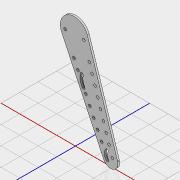
# Autodesk Inventor part: ЛЦМК.30000.30.00.02 Штанга
Saved by Autodesk Inventor 2021.2 (Build 252289000, 289)
## iProperties
Created: 2025-11-10
Part Number: ЛЦМК.30000.30.00.02 Штанга
Material: Типовые
Document SubType Name: Modeling
Designer: Захаров
Density: 1 g/cm^3
Appearance: По умолчанию
Mass: 8.66485 g
Surface Area: 67.4895 cm^2
Volume: 8.66485 cm^3
Author: Захаров
Autodesk Inventor part; units mm, degrees
ref_plane "YZ Plane" through (0, 0, 0) normal (1, 0, 0) x (0, 1, 0)
ref_plane "XZ Plane" through (0, 0, 0) normal (0, 1, 0) x (-1, 0, 0)
ref_plane "XY Plane" through (0, 0, 0) normal (0, 0, 1) x (1, 0, 0)
sketch "Эскиз1" plane through (0, 0, 0) normal (0, 0, 1) x (1, 0, 0)
  line L0 (15, -22.25) -> (15, 22.25) projected
  line L1 (15, 22.25) -> (-20, 22.25) projected
  line L2 (-20, 22.25) -> (-20, -22.25) projected
  line L3 (-20, -22.25) -> (15, -22.25) projected
  circle A0 centre (8.763, 2.3275) radius 1.5 projected
  circle A1 centre (8.763, 7.3275) radius 1.5 projected
  circle A2 centre (-11.237, -7.6725) radius 1.5 projected
  circle A3 centre (-11.237, -2.6725) radius 1.5 projected
  circle A4 centre (8.763, -2.6725) radius 1.5 projected
  circle A5 centre (8.763, -7.6725) radius 1.5 projected
  circle A6 centre (-11.237, 2.3275) radius 1.5 projected
  circle A7 centre (-11.237, 7.3275) radius 1.5 projected
  line L4 (-25, 92.25) -> (-62.0049, 92.25) projected
  line L5 (-103.637, 92.25) -> (-67.893, 92.25) projected
  circle A8 centre (-49, 104.25) radius 1.5 projected
  circle A9 centre (-42, 104.25) radius 1.5 projected
  circle A10 centre (-35, 104.25) radius 1.5 projected
  circle A11 centre (-35, 111.25) radius 1.5 projected
  circle A12 centre (-42, 118.25) radius 1.5 projected
  circle A13 centre (-49, 118.25) radius 1.5 projected
  circle A14 centre (-49, 111.25) radius 1.5 projected
  circle A15 centre (-35, 118.25) radius 1.5 projected
  circle A16 centre (-42, 111.25) radius 1.5 projected
  circle A17 centre (-42, 97.25) radius 1.5 projected
  circle A18 centre (-35, 97.25) radius 1.5 projected
  circle A19 centre (-49, 97.25) radius 1.5 projected
  line L6 (-25, 92.25) -> (-62.0049, 92.25) projected
  line L7 (-25, 95.25) -> (-25, 92.25) projected
  line L8 (-20, 95.25) -> (-25, 95.25) projected
  line L9 (-20, 95.25) -> (-20, 123.25) projected
  line L10 (-28, 123.25) -> (-20, 123.25) projected
  line L11 (-28, 129.25) -> (-28, 123.25) projected
  line L12 (-28, 129.25) -> (-62.0049, 129.25) projected
  line L13 (-62.0049, 92.25) -> (-62.0049, 129.25) projected
  line L14 (-5.1452, 11.625) -> (-40, 100) construction
  arc A20 (-32.5697, 102.9649) -> (-47.4303, 97.0351) centre (-40, 100) ccw
  line L15 (-5.1452, 11.625) -> (-22.5726, 55.8125) construction
  arc A21 (-13.8135, 8.0713) -> (-4.3725, 15.1785) centre (-0.8009, 0.6099) ccw
  line L16 (12.7625, 7.0157) -> (-32.7662, 103.4164)
  line L17 (-47.6184, 97.5588) -> (-15.0854, -3.9674)
  point P0 (0, 0)
  point P1 (-13.8589, 33.7187)
  point P2 (-33.6095, 104.8127)
  point P3 (-34.2206, 105.5316)
  point P4 (-47.7749, 98.1155)
  point P5 (-47.5011, 97.1926)
  dimension "d0" = 8
  dimension "d1" = 95
  dimension "d2" = 100
  dimension "d3" = 40
  dimension "d4" = 15
  constraints: 12 end point, 8 point on circle, 4 tangent, 2 centre point, 2 midpoint, 1 point on line
  measures "d0" radius of A20
  measures "d1" distance of L14.start L14.end
  measures "d2" vertical distance of point (0, 0) L14.end
  measures "d3" horizontal distance of point (0, 0) L14.end
  measures "d4" radius of A21
extrude "Выдавливание1" add sketch "Эскиз1" along normal blind 2 contours L16 A21 L17 L2 L1 | L1 L2 L17 L4 L16 | L4 L17 A19 A20 A10 L16 | A20 A10 | A10 A20 | A1 | A2 | A3 | A4 | A5 | A7 | A9
sketch "Эскиз2" plane through (0, 0, 2) normal (0, 0, 1) x (1, 0, 0)
  circle A0 centre (-38.5661, 86.5462) radius 1.5
  line L0 (-47.5011, 97.1926) -> (-15.0854, -3.9674) projected
  circle A1 centre (-35.5146, 77.0232) radius 1.5
  circle A2 centre (-32.463, 67.5001) radius 1.5
  circle A3 centre (-29.4114, 57.9771) radius 1.5
  circle A4 centre (-26.3599, 48.4541) radius 1.5
  circle A5 centre (-23.3083, 38.9311) radius 1.5
  circle A6 centre (-20.2568, 29.408) radius 1.5
  circle A7 centre (-17.2052, 19.885) radius 1.5
  circle A8 centre (-42, 97.25) radius 1.5 projected
  circle A9 centre (-11.237, 2.3275) radius 1.5 projected
  point P0 (0, 0)
  dimension "d7" = 3
  dimension "d10" = 10
  dimension "d17" = 5.2562
  dimension "d18" = 5.26
  constraints: 8 centre point, 15 other
  measures "d7" diameter of A0
  measures "d10" distance of A0.centre A1.centre
  measures "d17" distance from line of L0 A8.centre
  measures "d18" distance from line of L0 A0.centre
extrude "Выдавливание2" cut sketch "Эскиз2" against normal blind 3 contours A0 | A1 | A2 | A3 | A4 | A5 | A6 | A7
sketch "Эскиз3" plane through (0, 0, 2) normal (0, 0, 1) x (1, 0, 0)
  circle A0 centre (-35, 97.25) radius 1.5 projected
  line L0 (12.7625, 7.0157) -> (-32.7662, 103.4164) projected
  circle A1 centre (-30.5318, 87.7899) radius 1.5
  circle A2 centre (-26.2613, 78.7476) radius 1.5
  circle A3 centre (-21.9908, 69.7054) radius 1.5
  circle A4 centre (-17.7202, 60.6631) radius 1.5
  circle A5 centre (-13.4497, 51.6208) radius 1.5
  circle A6 centre (-9.1792, 42.5786) radius 1.5
  circle A7 centre (-4.9086, 33.5363) radius 1.5
  circle A8 centre (-0.6381, 24.494) radius 1.5
  point P0 (0, 0)
  dimension "d19" = 3
  dimension "d20" = 4.6533
  dimension "d21" = 4.653
  dimension "d24" = 10
  constraints: 8 centre point, 15 other
  measures "d19" diameter of A1
  measures "d20" distance from line of L0 A0.centre
  measures "d21" distance from line of L0 A1.centre
  measures "d24" distance of A1.centre A2.centre
extrude "Выдавливание3" cut sketch "Эскиз3" against normal blind 3 contours A1 | A2 | A3 | A4 | A5 | A6 | A7 | A8
sketch "Эскиз4" plane through (0, 0, 0) normal (0, 0, -1) x (-1, 0, 0)
  circle A0 centre (42, 97.25) radius 1.5 projected
  circle A1 centre (35, 97.25) radius 1.5 construction
  arc A2 (35, 97.25) -> (36.2942, 93.1949) centre (42, 97.25) ccw construction
  arc A3 (33.5, 97.25) -> (35.0715, 92.326) centre (42, 97.25) ccw
  arc A4 (36.5, 97.25) -> (37.5169, 94.0639) centre (42, 97.25) ccw
  arc A5 (36.5, 97.25) -> (33.5, 97.25) centre (35, 97.25) ccw construction
  arc A6 (35.0715, 92.326) -> (37.5169, 94.0639) centre (36.2942, 93.1949) ccw
  arc A7 (36.7604, 101.8918) -> (35.0715, 96.252) centre (42, 97.25) ccw construction
  arc A8 (35.6376, 102.8865) -> (33.5868, 96.0382) centre (42, 97.25) ccw
  arc A9 (37.8832, 100.8971) -> (36.5562, 96.4659) centre (42, 97.25) ccw
  arc A10 (37.8832, 100.8971) -> (35.6376, 102.8865) centre (36.7604, 101.8918) ccw
  arc A11 (33.5868, 96.0382) -> (36.5562, 96.4659) centre (35.0715, 96.252) ccw construction
  point P0 (0, 0)
  constraints: 21 point on circle, 10 centre point, 8 tangent, 2 coincident, 2 concentric
extrude "Выдавливание4" cut sketch "Эскиз4" against normal blind 3 contours A8 A10 A9 A4 A6 A3
sketch "Эскиз5" plane through (0, 0, 2) normal (0, 0, 1) x (1, 0, 0)
  circle A0 centre (-42, 97.25) radius 1.5 projected
  circle A1 centre (-11.237, 2.3275) radius 1.5 projected
  circle A2 centre (8.763, 2.3275) radius 1.5 projected
  arc A3 (-15.0854, -3.9674) -> (12.7625, 7.0157) centre (-0.8009, 0.6099) ccw projected
  line L0 (12.7625, 7.0157) -> (-32.7662, 103.4164) projected
  arc A4 (-32.7662, 103.4164) -> (-33.6095, 104.8127) centre (-40, 100) ccw projected
  arc A5 (-33.6095, 104.8127) -> (-34.2206, 105.5316) centre (-35, 104.25) ccw projected
  arc A6 (-34.2206, 105.5316) -> (-47.7749, 98.1155) centre (-40, 100) ccw projected
  arc A7 (-47.5011, 97.1926) -> (-47.7749, 98.1155) centre (-49, 97.25) ccw projected
  line L1 (-47.5011, 97.1926) -> (-15.0854, -3.9674) projected
  circle A8 centre (-17.2052, 19.885) radius 1.5 projected
  circle A9 centre (-23.3083, 38.9311) radius 1.5 projected
  circle A10 centre (-38.5661, 86.5462) radius 1.5 projected
  circle A11 centre (-32.463, 67.5001) radius 1.5 projected
  circle A12 centre (-29.4114, 57.9771) radius 1.5 projected
  circle A13 centre (-35.5146, 77.0232) radius 1.5 projected
  circle A14 centre (-20.2568, 29.408) radius 1.5 projected
  circle A15 centre (-26.3599, 48.4541) radius 1.5 projected
  circle A16 centre (-0.6381, 24.494) radius 1.5 projected
  circle A17 centre (-26.2613, 78.7476) radius 1.5 projected
  circle A18 centre (-4.9086, 33.5363) radius 1.5 projected
  circle A19 centre (-13.4497, 51.6208) radius 1.5 projected
  circle A20 centre (-17.7202, 60.6631) radius 1.5 projected
  circle A21 centre (-9.1792, 42.5786) radius 1.5 projected
  circle A22 centre (-30.5318, 87.7899) radius 1.5 projected
  circle A23 centre (-21.9908, 69.7054) radius 1.5 projected
  circle A24 centre (-23.3083, 38.9311) radius 1.5 projected
  circle A25 centre (-9.1792, 42.5786) radius 1.5 projected
  arc A26 (-9.149, 35.4026) -> (-9.1792, 42.5786) centre (-23.3083, 38.9311) ccw construction
  arc A27 (-7.6935, 35.0399) -> (-7.7268, 42.9535) centre (-23.3083, 38.9311) ccw
  arc A28 (-10.6045, 35.7653) -> (-10.6316, 42.2036) centre (-23.3083, 38.9311) ccw
  arc A29 (-10.6045, 35.7653) -> (-7.6935, 35.0399) centre (-9.149, 35.4026) ccw
  arc A30 (-7.7268, 42.9535) -> (-10.6316, 42.2036) centre (-9.1792, 42.5786) ccw
  arc A31 (-9.1792, 42.5786) -> (-11.0829, 46.8983) centre (-23.3083, 38.9311) ccw construction
  arc A32 (-7.7268, 42.9535) -> (-9.8263, 47.7173) centre (-23.3083, 38.9311) ccw
  arc A33 (-10.6316, 42.2036) -> (-12.3396, 46.0794) centre (-23.3083, 38.9311) ccw
  arc A34 (-10.6316, 42.2036) -> (-7.7268, 42.9535) centre (-9.1792, 42.5786) ccw
  arc A35 (-9.8263, 47.7173) -> (-12.3396, 46.0794) centre (-11.0829, 46.8983) ccw
  point P0 (0, 0)
  point P1 (-10.6316, 42.2036)
  point P2 (-10.6316, 42.2036)
  point P3 (-10.6316, 42.2036)
  point P4 (-7.7268, 42.9535)
  point P5 (-7.7268, 42.9535)
  point P6 (-7.7268, 42.9535)
  constraints: 20 point on circle, 10 centre point, 8 tangent, 2 coincident
extrude "Выдавливание5" cut sketch "Эскиз5" against normal blind 3 contours A21 A27 A29 A28 | A21 A33 A35 A32
